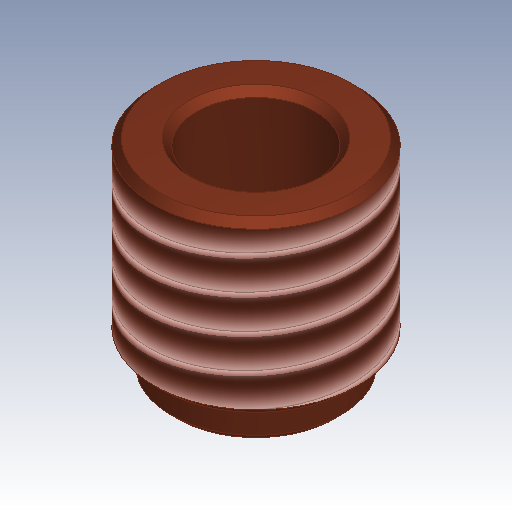
# Autodesk Inventor part: BT004_huenin20_23
Saved by Autodesk Inventor 2023.3 (Build 273359000, 359)
## iProperties
Company: HTBLA Kaindorf
RuleStatus: InUse
Created: 2023-08-12
Part Number: BT004_huenin20_23
Project: Fiberprinter-Hotend
Material: Kupfer
Description: Heatbreak_thread
Document SubType Name: Modeling
Designer: huenin20
Density: 8.94 g/cm^3
Appearance: Kupfer - satiniert
Mass: 0.998847 g
Surface Area: 2.11477 cm^2
Volume: 0.111728 cm^3
AfterDocNew0: iProperties-Editor_aufrufen
Author: nicob
Keywords: 2023
Autodesk Inventor part; units mm, degrees
ref_plane "YZ Plane" through (0, 0, 0) normal (1, 0, 0) x (0, 1, 0)
ref_plane "XZ Plane" through (0, 0, 0) normal (0, 1, 0) x (-1, 0, 0)
ref_plane "XY Plane" through (0, 0, 0) normal (0, 0, 1) x (1, 0, 0)
sketch "Skizze3" plane through (0, 0, 0) normal (1, 0, 0) x (0, 1, 0)
  line L0 (0, 0) -> (0, 9.4008)
  line L1 (-1, 0) -> (-1, 1.5)
  line L2 (-1, 1.5) -> (-1.75, 1.5)
  line L3 (-1.75, 1.5) -> (-1.75, 6)
  line L4 (-1.75, 6) -> (-3, 6)
  line L5 (-2.5, 0) -> (0, 0)
  line L6 (-3, 6) -> (-3, 1)
  line L7 (-3, 1) -> (-2.5, 1)
  line L8 (-2.5, 1) -> (-2.5, 0)
  dimension "d4" = 2
  dimension "d5" = 1.5
  dimension "d6" = 3.5
  dimension "d8" = 5
  dimension "d9" = 6
  dimension "d10" = 1
  dimension "d11" = 6
  constraints: 18 end point, 5 perpendicular, 3 vertical
  measures "d4" diameter of L1 L0
  measures "d5" distance between parallel lines of L5 L2
  measures "d6" diameter of L3 L0
  measures "d8" diameter of L8 L0
  measures "d9" diameter of L6 L0
  measures "d10" distance of L7.end L5.start
  measures "d11" distance between parallel lines of L5 L4
revolve "Umdrehung1" add sketch "Skizze3" angle 360 about axis through (0, 0, 0) along (0, 0, 1)
chamfer "Fase1" distance 0.2 angle 45 4 edges at (0, 1.75, 6) (0, 2.5, 0) (0, 3, 1) (0, 3, 6)
thread "Gewinde2" size "M6x1" class "6g" standard "ISO Metric profile" length 5
